Autodesk Inventor part; units mm, degrees
(part 2 of 2)
  spline S24 degree 3 poles (-2.2615, 80.5172) (-2.1729, 80.4485) (-1.9959, 80.3111) (-1.7411, 80.0916) (-1.5366, 79.9001) (-1.379, 79.7408) (-1.2639, 79.6183) (-1.1529, 79.4921) (-1.0079, 79.3211) (-0.9013, 79.1554) (-0.7866, 79.0322) (-0.7323, 78.9876) (-0.6853, 78.9569) (-0.6478, 78.9379) (-0.6091, 78.9214) (-0.5689, 78.909) (-0.5276, 78.9009) (-0.4857, 78.8971) (-0.4436, 78.8966) (-0.402, 78.903) (-0.3606, 78.9107) (-0.3079, 78.9303) (-0.2436, 78.958) (-0.1785, 78.9835) (-0.1272, 79.0065) (-0.0924, 79.0302) (-0.0583, 79.0548) (-0.0286, 79.0848) (-0.0015, 79.1169) (0.0221, 79.1518) (0.042, 79.1888) (0.058, 79.2277) (0.0713, 79.2677) (0.0832, 79.3225) (0.0904, 79.3923) (0.0854, 79.5606) (0.0448, 79.7534) (0.0277, 79.977) (0.018, 80.1448) (0.0138, 80.3128) (0.0139, 80.5369) (0.0248, 80.8169) (0.0517, 81.1521) (0.0811, 81.3743) (0.0958, 81.4854) knots 0 0 0 0 0.033613 0.067227 0.100839 0.117647 0.134454 0.151261 0.168068 0.201677 0.210077 0.218473 0.222676 0.226878 0.231076 0.235279 0.239479 0.24368 0.247882 0.252083 0.256283 0.260485 0.268889 0.277292 0.281494 0.285694 0.289895 0.294097 0.298298 0.302498 0.306701 0.310899 0.315101 0.319304 0.3277 0.3361 0.369709 0.386516 0.403323 0.420131 0.436938 0.470551 0.504164 0.537777 0.537777 0.537777 0.537777 projected
  arc A24 (-2.2615, 80.5172) -> (-2.9354, 80.1729) centre (6.5, 62.5385) ccw projected
  spline S25 degree 3 poles (-5.1012, 78.8299) (-5.0026, 78.7768) (-4.8053, 78.6704) (-4.5179, 78.4958) (-4.2846, 78.3406) (-4.1029, 78.2094) (-3.9692, 78.1075) (-3.839, 78.0012) (-3.6678, 77.8564) (-3.5354, 77.7105) (-3.4019, 77.6079) (-3.3411, 77.5728) (-3.2897, 77.5503) (-3.2496, 77.5377) (-3.2087, 77.5278) (-3.167, 77.5223) (-3.1249, 77.521) (-3.083, 77.5242) (-3.0413, 77.5306) (-3.0013, 77.5438) (-2.9618, 77.5582) (-2.9131, 77.5862) (-2.8542, 77.6241) (-2.7941, 77.66) (-2.7474, 77.6911) (-2.7169, 77.7202) (-2.6873, 77.7501) (-2.663, 77.7846) (-2.6416, 77.8207) (-2.624, 77.859) (-2.6104, 77.8988) (-2.6011, 77.9398) (-2.5946, 77.9814) (-2.5919, 78.0374) (-2.5962, 78.1075) (-2.6288, 78.2727) (-2.7006, 78.4562) (-2.7543, 78.6738) (-2.7915, 78.8377) (-2.8233, 79.0028) (-2.8601, 79.2239) (-2.8954, 79.5018) (-2.924, 79.8369) (-2.9316, 80.0609) (-2.9354, 80.1729) knots 0 0 0 0 0.033613 0.067227 0.100839 0.117647 0.134454 0.151261 0.168068 0.201677 0.210077 0.218473 0.222676 0.226878 0.231076 0.235279 0.239479 0.24368 0.247882 0.252083 0.256283 0.260485 0.268889 0.277292 0.281494 0.285694 0.289895 0.294097 0.298298 0.302498 0.306701 0.310899 0.315101 0.319304 0.3277 0.3361 0.369709 0.386516 0.403323 0.420131 0.436938 0.470551 0.504164 0.537777 0.537777 0.537777 0.537777 projected
  arc A25 (-5.1012, 78.8299) -> (-5.7093, 78.3793) centre (6.5, 62.5385) ccw projected
  spline S26 degree 3 poles (-7.6244, 76.6983) (-7.5184, 76.662) (-7.3063, 76.5896) (-6.9941, 76.4647) (-6.7384, 76.35) (-6.5377, 76.2504) (-6.389, 76.1719) (-6.243, 76.0886) (-6.0504, 75.9739) (-5.8958, 75.8518) (-5.7472, 75.7725) (-5.6814, 75.748) (-5.6271, 75.7342) (-5.5854, 75.7284) (-5.5434, 75.7254) (-5.5014, 75.7268) (-5.4597, 75.7324) (-5.4188, 75.7425) (-5.3788, 75.7557) (-5.3416, 75.7753) (-5.3049, 75.796) (-5.2615, 75.8317) (-5.2097, 75.8787) (-5.1563, 75.924) (-5.1153, 75.9624) (-5.09, 75.9961) (-5.0658, 76.0305) (-5.0475, 76.0684) (-5.0322, 76.1076) (-5.0212, 76.1483) (-5.0144, 76.1898) (-5.0119, 76.2318) (-5.0123, 76.2738) (-5.0189, 76.3295) (-5.0347, 76.398) (-5.0941, 76.5555) (-5.1951, 76.7247) (-5.2839, 76.9306) (-5.3476, 77.0861) (-5.4061, 77.2437) (-5.4788, 77.4557) (-5.5594, 77.724) (-5.6427, 78.0498) (-5.6871, 78.2695) (-5.7093, 78.3793) knots 0 0 0 0 0.033613 0.067227 0.100839 0.117647 0.134454 0.151261 0.168068 0.201677 0.210077 0.218473 0.222676 0.226878 0.231076 0.235279 0.239479 0.24368 0.247882 0.252083 0.256283 0.260485 0.268889 0.277292 0.281494 0.285694 0.289895 0.294097 0.298298 0.302498 0.306701 0.310899 0.315101 0.319304 0.3277 0.3361 0.369709 0.386516 0.403323 0.420131 0.436938 0.470551 0.504164 0.537777 0.537777 0.537777 0.537777 projected
  arc A26 (-7.6244, 76.6983) -> (-8.1501, 76.1537) centre (6.5, 62.5385) ccw projected
  spline S27 degree 3 poles (-9.7624, 74.1803) (-9.6519, 74.162) (-9.4308, 74.1255) (-9.1022, 74.0537) (-8.8312, 73.9826) (-8.6168, 73.9175) (-8.4572, 73.8645) (-8.2995, 73.8064) (-8.0906, 73.7249) (-7.918, 73.63) (-7.7585, 73.5762) (-7.6895, 73.5628) (-7.6336, 73.5582) (-7.5916, 73.5593) (-7.5497, 73.5633) (-7.5084, 73.5715) (-7.4682, 73.584) (-7.4296, 73.6006) (-7.3923, 73.6203) (-7.3588, 73.6457) (-7.326, 73.6722) (-7.2891, 73.7145) (-7.2457, 73.7694) (-7.2005, 73.8229) (-7.1664, 73.8675) (-7.147, 73.9049) (-7.1288, 73.9428) (-7.1169, 73.9833) (-7.1084, 74.0244) (-7.1042, 74.0663) (-7.1043, 74.1084) (-7.1088, 74.1502) (-7.1161, 74.1916) (-7.1317, 74.2455) (-7.1586, 74.3104) (-7.2431, 74.456) (-7.3706, 74.6063) (-7.492, 74.7947) (-7.5804, 74.9376) (-7.6641, 75.0834) (-7.7707, 75.2806) (-7.8944, 75.532) (-8.0302, 75.8396) (-8.1101, 76.049) (-8.1501, 76.1537) knots 0 0 0 0 0.033613 0.067227 0.100839 0.117647 0.134454 0.151261 0.168068 0.201677 0.210077 0.218473 0.222676 0.226878 0.231076 0.235279 0.239479 0.24368 0.247882 0.252083 0.256283 0.260485 0.268889 0.277292 0.281494 0.285694 0.289895 0.294097 0.298298 0.302498 0.306701 0.310899 0.315101 0.319304 0.3277 0.3361 0.369709 0.386516 0.403323 0.420131 0.436938 0.470551 0.504164 0.537777 0.537777 0.537777 0.537777 projected
  arc A27 (-9.7624, 74.1803) -> (-10.1913, 73.5567) centre (6.5, 62.5385) ccw projected
  spline S28 degree 3 poles (-11.4568, 71.3448) (-11.3448, 71.345) (-11.1206, 71.3453) (-10.7848, 71.3286) (-10.5057, 71.3031) (-10.2835, 71.2742) (-10.1174, 71.2482) (-9.9523, 71.2168) (-9.7329, 71.1708) (-9.547, 71.1056) (-9.3808, 71.0788) (-9.3105, 71.0769) (-9.2546, 71.0816) (-9.2133, 71.0896) (-9.1727, 71.1004) (-9.1334, 71.1153) (-9.0957, 71.1343) (-9.0604, 71.157) (-9.0268, 71.1825) (-8.9979, 71.2131) (-8.97, 71.2446) (-8.9405, 71.2924) (-8.9068, 71.3538) (-8.871, 71.4139) (-8.8447, 71.4636) (-8.8317, 71.5036) (-8.82, 71.544) (-8.815, 71.5859) (-8.8133, 71.6279) (-8.8161, 71.6699) (-8.8231, 71.7114) (-8.8344, 71.7519) (-8.8484, 71.7916) (-8.8727, 71.8421) (-8.9099, 71.9017) (-9.0172, 72.0314) (-9.1677, 72.1586) (-9.3185, 72.3245) (-9.4292, 72.451) (-9.5358, 72.581) (-9.6734, 72.7579) (-9.8367, 72.9856) (-10.0213, 73.2666) (-10.1346, 73.46) (-10.1913, 73.5567) knots 0 0 0 0 0.033613 0.067227 0.100839 0.117647 0.134454 0.151261 0.168068 0.201677 0.210077 0.218473 0.222676 0.226878 0.231076 0.235279 0.239479 0.24368 0.247882 0.252083 0.256283 0.260485 0.268889 0.277292 0.281494 0.285694 0.289895 0.294097 0.298298 0.302498 0.306701 0.310899 0.315101 0.319304 0.3277 0.3361 0.369709 0.386516 0.403323 0.420131 0.436938 0.470551 0.504164 0.537777 0.537777 0.537777 0.537777 projected
  arc A28 (-11.4568, 71.3448) -> (-11.7772, 70.6591) centre (6.5, 62.5385) ccw projected
  spline S29 degree 3 poles (-12.6614, 68.2691) (-12.5509, 68.2877) (-12.3299, 68.325) (-11.9959, 68.3637) (-11.7164, 68.3845) (-11.4925, 68.3926) (-11.3244, 68.3943) (-11.1563, 68.3905) (-10.9323, 68.3813) (-10.7382, 68.3475) (-10.5699, 68.3484) (-10.5003, 68.3582) (-10.4459, 68.372) (-10.4065, 68.3867) (-10.3682, 68.404) (-10.3319, 68.4252) (-10.2979, 68.4501) (-10.2667, 68.4783) (-10.2378, 68.509) (-10.2144, 68.5439) (-10.192, 68.5796) (-10.1708, 68.6316) (-10.1476, 68.6977) (-10.1222, 68.7629) (-10.1045, 68.8162) (-10.0982, 68.8578) (-10.0933, 68.8996) (-10.0953, 68.9417) (-10.1005, 68.9834) (-10.1102, 69.0244) (-10.1239, 69.0642) (-10.1417, 69.1023) (-10.1621, 69.1391) (-10.1944, 69.185) (-10.2409, 69.2376) (-10.3681, 69.3479) (-10.5374, 69.4486) (-10.7135, 69.5874) (-10.8435, 69.6939) (-10.97, 69.8046) (-11.1348, 69.9565) (-11.3334, 70.1541) (-11.5618, 70.401) (-11.7054, 70.5731) (-11.7772, 70.6591) knots 0 0 0 0 0.033613 0.067227 0.100839 0.117647 0.134454 0.151261 0.168068 0.201677 0.210077 0.218473 0.222676 0.226878 0.231076 0.235279 0.239479 0.24368 0.247882 0.252083 0.256283 0.260485 0.268889 0.277292 0.281494 0.285694 0.289895 0.294097 0.298298 0.302498 0.306701 0.310899 0.315101 0.319304 0.3277 0.3361 0.369709 0.386516 0.403323 0.420131 0.436938 0.470551 0.504164 0.537777 0.537777 0.537777 0.537777 projected
  arc A29 (-12.6614, 68.2691) -> (-12.8645, 67.5401) centre (6.5, 62.5385) ccw projected
  spline S30 degree 3 poles (-13.3433, 65.0371) (-13.2374, 65.0737) (-13.0255, 65.1467) (-12.7024, 65.2399) (-12.4302, 65.3065) (-12.2106, 65.3513) (-12.0451, 65.3806) (-11.8787, 65.4045) (-11.6563, 65.4323) (-11.4592, 65.431) (-11.2933, 65.4596) (-11.2263, 65.4806) (-11.175, 65.5032) (-11.1385, 65.5242) (-11.1036, 65.5476) (-11.0712, 65.5745) (-11.0418, 65.6046) (-11.0157, 65.6376) (-10.9923, 65.6726) (-10.9749, 65.7109) (-10.9587, 65.7498) (-10.9463, 65.8046) (-10.9343, 65.8736) (-10.92, 65.9421) (-10.9113, 65.9976) (-10.912, 66.0397) (-10.914, 66.0817) (-10.9229, 66.1229) (-10.9349, 66.1632) (-10.9512, 66.202) (-10.9713, 66.239) (-10.9951, 66.2736) (-11.0213, 66.3066) (-11.0607, 66.3465) (-11.1152, 66.3908) (-11.2588, 66.4786) (-11.4424, 66.5501) (-11.6389, 66.658) (-11.7847, 66.7417) (-11.9277, 66.83) (-12.1153, 66.9527) (-12.3437, 67.115) (-12.6096, 67.3209) (-12.7795, 67.467) (-12.8645, 67.5401) knots 0 0 0 0 0.033613 0.067227 0.100839 0.117647 0.134454 0.151261 0.168068 0.201677 0.210077 0.218473 0.222676 0.226878 0.231076 0.235279 0.239479 0.24368 0.247882 0.252083 0.256283 0.260485 0.268889 0.277292 0.281494 0.285694 0.289895 0.294097 0.298298 0.302498 0.306701 0.310899 0.315101 0.319304 0.3277 0.3361 0.369709 0.386516 0.403323 0.420131 0.436938 0.470551 0.504164 0.537777 0.537777 0.537777 0.537777 projected
  arc A30 (-13.3433, 65.0371) -> (-13.4236, 64.2845) centre (6.5, 62.5385) ccw projected
  spline S31 degree 3 poles (-13.4839, 61.7369) (-13.3855, 61.7904) (-13.1885, 61.8974) (-12.8852, 62.0425) (-12.6276, 62.1529) (-12.4184, 62.2332) (-12.26, 62.2894) (-12.0998, 62.3404) (-11.885, 62.4044) (-11.6904, 62.4355) (-11.5315, 62.4911) (-11.4688, 62.5229) (-11.4219, 62.5536) (-11.3894, 62.5803) (-11.3588, 62.6091) (-11.3313, 62.641) (-11.3072, 62.6755) (-11.2869, 62.7123) (-11.2696, 62.7507) (-11.2587, 62.7914) (-11.2491, 62.8324) (-11.246, 62.8885) (-11.2455, 62.9585) (-11.2427, 63.0284) (-11.2432, 63.0846) (-11.2508, 63.126) (-11.2597, 63.1671) (-11.2752, 63.2063) (-11.2937, 63.2441) (-11.3162, 63.2797) (-11.3421, 63.3128) (-11.3713, 63.3431) (-11.4025, 63.3713) (-11.448, 63.4042) (-11.509, 63.4389) (-11.6652, 63.5019) (-11.858, 63.5422) (-12.0696, 63.6163) (-12.2272, 63.6748) (-12.3828, 63.7384) (-12.588, 63.8285) (-12.84, 63.951) (-13.1361, 64.1103) (-13.3278, 64.2265) (-13.4236, 64.2845) knots 0 0 0 0 0.033613 0.067227 0.100839 0.117647 0.134454 0.151261 0.168068 0.201677 0.210077 0.218473 0.222676 0.226878 0.231076 0.235279 0.239479 0.24368 0.247882 0.252083 0.256283 0.260485 0.268889 0.277292 0.281494 0.285694 0.289895 0.294097 0.298298 0.302498 0.306701 0.310899 0.315101 0.319304 0.3277 0.3361 0.369709 0.386516 0.403323 0.420131 0.436938 0.470551 0.504164 0.537777 0.537777 0.537777 0.537777 projected
  arc A31 (-13.4839, 61.7369) -> (-13.4393, 60.9814) centre (6.5, 62.5385) ccw projected
  spline S32 degree 3 poles (-13.0795, 58.4586) (-12.9911, 58.5276) (-12.8145, 58.6655) (-12.5391, 58.8586) (-12.3033, 59.0099) (-12.1101, 59.1235) (-11.9631, 59.205) (-11.8135, 59.2817) (-11.6121, 59.3802) (-11.4254, 59.4429) (-11.2777, 59.5238) (-11.2212, 59.5655) (-11.1799, 59.6035) (-11.1523, 59.6352) (-11.1268, 59.6687) (-11.105, 59.7046) (-11.0869, 59.7426) (-11.0729, 59.7823) (-11.0621, 59.8231) (-11.0581, 59.865) (-11.0554, 59.907) (-11.0616, 59.9628) (-11.0726, 60.0319) (-11.0813, 60.1014) (-11.0911, 60.1567) (-11.1054, 60.1963) (-11.121, 60.2354) (-11.1427, 60.2715) (-11.1672, 60.3057) (-11.1952, 60.3371) (-11.2262, 60.3655) (-11.26, 60.3906) (-11.2954, 60.4133) (-11.3457, 60.4382) (-11.4116, 60.4624) (-11.576, 60.4989) (-11.7728, 60.5068) (-11.9937, 60.5451) (-12.1588, 60.5769) (-12.3227, 60.614) (-12.54, 60.6692) (-12.8087, 60.7485) (-13.127, 60.8569) (-13.3352, 60.9399) (-13.4393, 60.9814) knots 0 0 0 0 0.033613 0.067227 0.100839 0.117647 0.134454 0.151261 0.168068 0.201677 0.210077 0.218473 0.222676 0.226878 0.231076 0.235279 0.239479 0.24368 0.247882 0.252083 0.256283 0.260485 0.268889 0.277292 0.281494 0.285694 0.289895 0.294097 0.298298 0.302498 0.306701 0.310899 0.315101 0.319304 0.3277 0.3361 0.369709 0.386516 0.403323 0.420131 0.436938 0.470551 0.504164 0.537777 0.537777 0.537777 0.537777 projected
  arc A32 (-13.0795, 58.4586) -> (-12.9111, 57.7207) centre (6.5, 62.5385) ccw projected
  spline S33 degree 3 poles (-12.1409, 55.2916) (-12.0651, 55.3741) (-11.9136, 55.5393) (-11.6738, 55.775) (-11.466, 55.9631) (-11.2942, 56.107) (-11.1626, 56.2116) (-11.0277, 56.3118) (-10.8453, 56.4421) (-10.6714, 56.5347) (-10.5391, 56.6388) (-10.4902, 56.6892) (-10.4557, 56.7335) (-10.4337, 56.7693) (-10.4141, 56.8065) (-10.3984, 56.8456) (-10.3869, 56.8861) (-10.3796, 56.9275) (-10.3757, 56.9695) (-10.3786, 57.0114) (-10.3829, 57.0533) (-10.3981, 57.1074) (-10.4204, 57.1738) (-10.4404, 57.2408) (-10.4591, 57.2938) (-10.4798, 57.3305) (-10.5016, 57.3665) (-10.529, 57.3985) (-10.5587, 57.4282) (-10.5915, 57.4546) (-10.6268, 57.4775) (-10.6643, 57.4967) (-10.7029, 57.5132) (-10.7566, 57.5296) (-10.8256, 57.5426) (-10.9937, 57.5515) (-11.1892, 57.5269) (-11.4134, 57.5283) (-11.5814, 57.5325) (-11.7493, 57.5422) (-11.9726, 57.5608) (-12.2507, 57.5948) (-12.5826, 57.6493) (-12.8016, 57.6969) (-12.9111, 57.7207) knots 0 0 0 0 0.033613 0.067227 0.100839 0.117647 0.134454 0.151261 0.168068 0.201677 0.210077 0.218473 0.222676 0.226878 0.231076 0.235279 0.239479 0.24368 0.247882 0.252083 0.256283 0.260485 0.268889 0.277292 0.281494 0.285694 0.289895 0.294097 0.298298 0.302498 0.306701 0.310899 0.315101 0.319304 0.3277 0.3361 0.369709 0.386516 0.403323 0.420131 0.436938 0.470551 0.504164 0.537777 0.537777 0.537777 0.537777 projected
  arc A33 (-12.1409, 55.2916) -> (-11.8534, 54.5915) centre (6.5, 62.5385) ccw projected
  spline S34 degree 3 poles (-10.6939, 52.3222) (-10.6327, 52.4161) (-10.5104, 52.6039) (-10.3127, 52.8759) (-10.1387, 53.0956) (-9.993, 53.2658) (-9.8804, 53.3907) (-9.7638, 53.5117) (-9.6053, 53.6703) (-9.449, 53.7903) (-9.3356, 53.9148) (-9.2957, 53.9725) (-9.269, 54.0219) (-9.2531, 54.0608) (-9.2399, 54.1007) (-9.2309, 54.1418) (-9.2262, 54.1837) (-9.2259, 54.2257) (-9.2289, 54.2678) (-9.2387, 54.3087) (-9.2498, 54.3493) (-9.2737, 54.4001) (-9.3066, 54.4619) (-9.3374, 54.5248) (-9.3646, 54.5739) (-9.391, 54.6067) (-9.4184, 54.6387) (-9.4507, 54.6657) (-9.485, 54.6901) (-9.5216, 54.7108) (-9.5602, 54.7276) (-9.6003, 54.7403) (-9.6412, 54.7502) (-9.6968, 54.7575) (-9.767, 54.759) (-9.9343, 54.7401) (-10.1231, 54.6837) (-10.3445, 54.6482) (-10.5109, 54.6247) (-10.678, 54.6066) (-10.9014, 54.5882) (-11.1813, 54.5759) (-11.5176, 54.5751) (-11.7414, 54.586) (-11.8534, 54.5915) knots 0 0 0 0 0.033613 0.067227 0.100839 0.117647 0.134454 0.151261 0.168068 0.201677 0.210077 0.218473 0.222676 0.226878 0.231076 0.235279 0.239479 0.24368 0.247882 0.252083 0.256283 0.260485 0.268889 0.277292 0.281494 0.285694 0.289895 0.294097 0.298298 0.302498 0.306701 0.310899 0.315101 0.319304 0.3277 0.3361 0.369709 0.386516 0.403323 0.420131 0.436938 0.470551 0.504164 0.537777 0.537777 0.537777 0.537777 projected
  arc A34 (-10.6939, 52.3222) -> (-10.295, 51.679) centre (6.5, 62.5385) ccw projected
  spline S35 degree 3 poles (-8.7778, 49.6316) (-8.733, 49.7342) (-8.6432, 49.9396) (-8.493, 50.2405) (-8.3576, 50.4858) (-8.2418, 50.6777) (-8.1513, 50.8193) (-8.0562, 50.9579) (-7.926, 51.1404) (-7.7915, 51.2844) (-7.7003, 51.4259) (-7.6703, 51.4895) (-7.6522, 51.5425) (-7.6429, 51.5836) (-7.6365, 51.6251) (-7.6343, 51.6671) (-7.6366, 51.7092) (-7.6432, 51.7507) (-7.6531, 51.7917) (-7.6695, 51.8304) (-7.6871, 51.8687) (-7.7191, 51.9149) (-7.7617, 51.9704) (-7.8024, 52.0273) (-7.8373, 52.0714) (-7.8687, 52.0993) (-7.901, 52.1263) (-7.9374, 52.1477) (-7.9752, 52.1661) (-8.0147, 52.1805) (-8.0556, 52.1907) (-8.0972, 52.1966) (-8.1391, 52.1997) (-8.1952, 52.1978) (-8.2647, 52.1876) (-8.4266, 52.1415) (-8.6035, 52.0548) (-8.816, 51.9833) (-8.9763, 51.9327) (-9.1382, 51.8873) (-9.3555, 51.8324) (-9.6296, 51.7743) (-9.9611, 51.7181) (-10.1837, 51.692) (-10.295, 51.679) knots 0 0 0 0 0.033613 0.067227 0.100839 0.117647 0.134454 0.151261 0.168068 0.201677 0.210077 0.218473 0.222676 0.226878 0.231076 0.235279 0.239479 0.24368 0.247882 0.252083 0.256283 0.260485 0.268889 0.277292 0.281494 0.285694 0.289895 0.294097 0.298298 0.302498 0.306701 0.310899 0.315101 0.319304 0.3277 0.3361 0.369709 0.386516 0.403323 0.420131 0.436938 0.470551 0.504164 0.537777 0.537777 0.537777 0.537777 projected
  arc A35 (-8.7778, 49.6316) -> (-8.2785, 49.0628) centre (6.5, 62.5385) ccw projected
  spline S36 degree 3 poles (-6.445, 47.2929) (-6.4177, 47.4016) (-6.363, 47.619) (-6.2643, 47.9404) (-6.1711, 48.2047) (-6.0885, 48.413) (-6.0226, 48.5676) (-5.9516, 48.72) (-5.8532, 48.9214) (-5.7443, 49.0856) (-5.6775, 49.2402) (-5.6585, 49.3078) (-5.6493, 49.3631) (-5.6469, 49.4051) (-5.6474, 49.4472) (-5.6522, 49.489) (-5.6613, 49.5301) (-5.6747, 49.5699) (-5.6912, 49.6087) (-5.7137, 49.6443) (-5.7374, 49.6791) (-5.7765, 49.7194) (-5.8277, 49.7671) (-5.8772, 49.8166) (-5.9189, 49.8543) (-5.9545, 49.8767) (-5.9908, 49.898) (-6.0302, 49.9131) (-6.0705, 49.9251) (-6.1119, 49.9327) (-6.1539, 49.9361) (-6.1959, 49.935) (-6.2378, 49.9312) (-6.2927, 49.92) (-6.3596, 49.8986) (-6.5117, 49.8264) (-6.672, 49.7118) (-6.8698, 49.6063) (-7.0196, 49.53) (-7.1718, 49.4586) (-7.3771, 49.3687) (-7.6379, 49.2663) (-7.9556, 49.1563) (-8.1709, 49.0939) (-8.2785, 49.0628) knots 0 0 0 0 0.033613 0.067227 0.100839 0.117647 0.134454 0.151261 0.168068 0.201677 0.210077 0.218473 0.222676 0.226878 0.231076 0.235279 0.239479 0.24368 0.247882 0.252083 0.256283 0.260485 0.268889 0.277292 0.281494 0.285694 0.289895 0.294097 0.298298 0.302498 0.306701 0.310899 0.315101 0.319304 0.3277 0.3361 0.369709 0.386516 0.403323 0.420131 0.436938 0.470551 0.504164 0.537777 0.537777 0.537777 0.537777 projected
  arc A36 (-6.445, 47.2929) -> (-5.859, 46.8141) centre (6.5, 62.5385) ccw projected
  spline S37 degree 3 poles (-3.7592, 45.3702) (-3.7501, 45.4819) (-3.7319, 45.7053) (-3.6875, 46.0386) (-3.639, 46.3146) (-3.5919, 46.5337) (-3.5522, 46.697) (-3.5073, 46.859) (-3.4434, 47.0739) (-3.363, 47.2538) (-3.3226, 47.4172) (-3.3149, 47.487) (-3.315, 47.5431) (-3.3196, 47.5849) (-3.3269, 47.6263) (-3.3386, 47.6668) (-3.3543, 47.7058) (-3.3741, 47.7429) (-3.3967, 47.7785) (-3.4248, 47.8098) (-3.4539, 47.8402) (-3.4992, 47.8736) (-3.5575, 47.9122) (-3.6145, 47.9529) (-3.6618, 47.9832) (-3.7006, 47.9994) (-3.7399, 48.0145) (-3.7812, 48.0229) (-3.823, 48.0281) (-3.8651, 48.0288) (-3.907, 48.0252) (-3.9483, 48.0173) (-3.989, 48.0066) (-4.0413, 47.9865) (-4.1038, 47.9544) (-4.242, 47.8581) (-4.3812, 47.7187) (-4.5589, 47.5821) (-4.6941, 47.4822) (-4.8324, 47.3867) (-5.0201, 47.2643) (-5.2605, 47.1203) (-5.5558, 46.9595) (-5.7579, 46.8625) (-5.859, 46.8141) knots 0 0 0 0 0.033613 0.067227 0.100839 0.117647 0.134454 0.151261 0.168068 0.201677 0.210077 0.218473 0.222676 0.226878 0.231076 0.235279 0.239479 0.24368 0.247882 0.252083 0.256283 0.260485 0.268889 0.277292 0.281494 0.285694 0.289895 0.294097 0.298298 0.302498 0.306701 0.310899 0.315101 0.319304 0.3277 0.3361 0.369709 0.386516 0.403323 0.420131 0.436938 0.470551 0.504164 0.537777 0.537777 0.537777 0.537777 projected
  arc A37 (-3.7592, 45.3702) -> (-3.1023, 44.9943) centre (6.5, 62.5385) ccw projected
  circle A38 centre (6.5, 62.5385) radius 16 projected
  arc A39 (25.4036, 41.8198) -> (23.2102, 40.8992) centre (27.6407, 33.4167) ccw projected
  arc A40 (23.2102, 40.8992) -> (22.7103, 41.3835) centre (16.1803, 34.1432) ccw projected
  arc A41 (22.7103, 41.3835) -> (23.561, 43.6049) centre (15.0912, 45.5749) ccw projected
  arc A42 (23.561, 43.6049) -> (22.8672, 44.1074) centre (16.1803, 34.1432) ccw projected
  arc A43 (22.8672, 44.1074) -> (21.022, 42.606) centre (27.3812, 36.6749) ccw projected
  arc A44 (21.022, 42.606) -> (20.406, 42.9299) centre (16.1803, 34.1432) ccw projected
  arc A45 (20.406, 42.9299) -> (20.5964, 45.3011) centre (11.9147, 44.805) ccw projected
  arc A46 (20.5964, 45.3011) -> (19.7891, 45.5877) centre (16.1803, 34.1432) ccw projected
  arc A47 (19.7891, 45.5877) -> (18.4416, 43.6273) centre (26.2142, 39.728) ccw projected
  arc A48 (18.4416, 43.6273) -> (17.7593, 43.7645) centre (16.1803, 34.1432) ccw projected
  arc A49 (17.7593, 43.7645) -> (17.2739, 46.0932) centre (9.0837, 43.1713) ccw projected
  arc A50 (17.2739, 46.0932) -> (16.4186, 46.1408) centre (16.1803, 34.1432) ccw projected
  arc A51 (16.4186, 46.1408) -> (15.678, 43.8802) centre (24.2344, 42.3286) ccw projected
  arc A52 (15.678, 43.8802) -> (14.9847, 43.8196) centre (16.1803, 34.1432) ccw projected
  arc A53 (14.9847, 43.8196) -> (13.8629, 45.9173) centre (6.8276, 40.8063) ccw projected
  arc A54 (13.8629, 45.9173) -> (13.0289, 45.722) centre (16.1803, 34.1432) ccw projected
  arc A55 (13.0289, 45.722) -> (12.9551, 43.3443) centre (21.602, 44.2662) ccw projected
  arc A56 (12.9551, 43.3443) -> (12.307, 43.0908) centre (16.1803, 34.1432) ccw projected
  arc A57 (12.307, 43.0908) -> (10.6396, 44.7875) centre (5.3292, 37.9014) ccw projected
  arc A58 (10.6396, 44.7875) -> (9.8944, 44.3651) centre (16.1803, 34.1432) ccw projected
  arc A59 (9.8944, 44.3651) -> (10.4935, 42.063) centre (18.5304, 45.3836) ccw projected
  arc A60 (10.4935, 42.063) -> (9.943, 41.6371) centre (16.1803, 34.1432) ccw projected
  arc A61 (9.943, 41.6371) -> (7.8652, 42.7953) centre (4.71, 34.6921) ccw projected
  arc A62 (7.8652, 42.7953) -> (7.2692, 42.1801) centre (16.1803, 34.1432) ccw projected
  arc A63 (7.2692, 42.1801) -> (8.4926, 40.14) centre (15.2684, 45.5904) ccw projected
  arc A64 (8.4926, 40.14) -> (8.0844, 39.5763) centre (16.1803, 34.1432) ccw projected
  arc A65 (8.0844, 39.5763) -> (5.7645, 40.1022) centre (5.0199, 31.4383) ccw projected
  arc A66 (5.7645, 40.1022) -> (5.3659, 39.344) centre (16.1803, 34.1432) ccw projected
  arc A67 (5.3659, 39.344) -> (7.1145, 37.7312) centre (12.0803, 44.8698) ccw projected
  arc A68 (7.1145, 37.7312) -> (6.8816, 37.0753) centre (16.1803, 34.1432) ccw projected
  arc A69 (6.8816, 37.0753) -> (4.5075, 36.9264) centre (6.2341, 28.4036) ccw projected
  arc A70 (4.5075, 36.9264) -> (4.3387, 36.0865) centre (16.1803, 34.1432) ccw projected
  arc A71 (4.3387, 36.0865) -> (6.4709, 35.0318) centre (9.2244, 43.2802) ccw projected
  arc A72 (6.4709, 35.0318) -> (6.4322, 34.3368) centre (16.1803, 34.1432) ccw projected
  arc A73 (6.4322, 34.3368) -> (4.1962, 33.525) centre (8.254, 25.8339) ccw projected
  arc A74 (4.1962, 33.525) -> (4.2709, 32.6717) centre (16.1803, 34.1432) ccw projected
  arc A75 (4.2709, 32.6717) -> (6.6138, 32.2603) centre (6.9319, 40.9503) ccw projected
  arc A76 (6.6138, 32.2603) -> (6.7725, 31.5826) centre (16.1803, 34.1432) ccw projected
  arc A77 (6.7725, 31.5826) -> (4.8558, 30.1738) centre (10.916, 23.9374) ccw projected
  arc A78 (4.8558, 30.1738) -> (5.1679, 29.376) centre (16.1803, 34.1432) ccw projected
  arc A79 (5.1679, 29.376) -> (7.5318, 29.6414) centre (5.3888, 38.069) ccw projected
  arc A80 (7.5318, 29.6414) -> (7.875, 29.0359) centre (16.1803, 34.1432) ccw projected
  arc A81 (7.875, 29.0359) -> (6.4329, 27.1441) centre (14.0046, 22.8677) ccw projected
  arc A82 (6.4329, 27.1441) -> (6.957, 26.4665) centre (16.1803, 34.1432) ccw projected
  arc A83 (6.957, 26.4665) -> (9.1504, 27.3872) centre (4.7198, 34.8697) ccw projected
  arc A84 (9.1504, 27.3872) -> (9.6503, 26.9029) centre (16.1803, 34.1432) ccw projected
  arc A85 (9.6503, 26.9029) -> (8.7996, 24.6814) centre (17.2694, 22.7115) ccw projected
  arc A86 (8.7996, 24.6814) -> (9.4934, 24.179) centre (16.1803, 34.1432) ccw projected
  arc A87 (9.4934, 24.179) -> (11.3386, 25.6803) centre (4.9794, 31.6115) ccw projected
  arc A88 (11.3386, 25.6803) -> (11.9546, 25.3565) centre (16.1803, 34.1432) ccw projected
  arc A89 (11.9546, 25.3565) -> (11.7642, 22.9853) centre (20.4459, 23.4814) ccw projected
  arc A90 (11.7642, 22.9853) -> (12.5715, 22.6987) centre (16.1803, 34.1432) ccw projected
  arc A91 (12.5715, 22.6987) -> (13.919, 24.659) centre (6.1464, 28.5584) ccw projected
  arc A92 (13.919, 24.659) -> (14.6013, 24.5219) centre (16.1803, 34.1432) ccw projected
  arc A93 (14.6013, 24.5219) -> (15.0867, 22.1931) centre (23.2769, 25.115) ccw projected
  arc A94 (15.0867, 22.1931) -> (15.9419, 22.1455) centre (16.1803, 34.1432) ccw projected
  arc A95 (15.9419, 22.1455) -> (16.6826, 24.4061) centre (8.1262, 25.9577) ccw projected
  arc A96 (16.6826, 24.4061) -> (17.3759, 24.4668) centre (16.1803, 34.1432) ccw projected
  arc A97 (17.3759, 24.4668) -> (18.4977, 22.3691) centre (25.533, 27.4801) ccw projected
  arc A98 (18.4977, 22.3691) -> (19.3317, 22.5644) centre (16.1803, 34.1432) ccw projected
  arc A99 (19.3317, 22.5644) -> (19.4055, 24.942) centre (10.7586, 24.0202) ccw projected
  arc A100 (19.4055, 24.942) -> (20.0536, 25.1956) centre (16.1803, 34.1432) ccw projected
  arc A101 (20.0536, 25.1956) -> (21.721, 23.4989) centre (27.0313, 30.3849) ccw projected
  arc A102 (21.721, 23.4989) -> (22.4662, 23.9213) centre (16.1803, 34.1432) ccw projected
  arc A103 (22.4662, 23.9213) -> (21.8671, 26.2234) centre (13.8302, 22.9028) ccw projected
  arc A104 (21.8671, 26.2234) -> (22.4176, 26.6493) centre (16.1803, 34.1432) ccw projected
  arc A105 (22.4176, 26.6493) -> (24.4954, 25.491) centre (27.6506, 33.5943) ccw projected
  arc A106 (24.4954, 25.491) -> (25.0914, 26.1063) centre (16.1803, 34.1432) ccw projected
  arc A107 (25.0914, 26.1063) -> (23.868, 28.1463) centre (17.0922, 22.696) ccw projected
  arc A108 (23.868, 28.1463) -> (24.2762, 28.7101) centre (16.1803, 34.1432) ccw projected
  arc A109 (24.2762, 28.7101) -> (26.5961, 28.1841) centre (27.3406, 36.8481) ccw projected
  arc A110 (26.5961, 28.1841) -> (26.9947, 28.9424) centre (16.1803, 34.1432) ccw projected
  arc A111 (26.9947, 28.9424) -> (25.2461, 30.5551) centre (20.2803, 23.4166) ccw projected
  arc A112 (25.2461, 30.5551) -> (25.4789, 31.211) centre (16.1803, 34.1432) ccw projected
  arc A113 (25.4789, 31.211) -> (27.8531, 31.36) centre (26.1265, 39.8827) ccw projected
  arc A114 (27.8531, 31.36) -> (28.0219, 32.1998) centre (16.1803, 34.1432) ccw projected
  arc A115 (28.0219, 32.1998) -> (25.8897, 33.2546) centre (23.1362, 25.0062) ccw projected
  arc A116 (25.8897, 33.2546) -> (25.9284, 33.9495) centre (16.1803, 34.1432) ccw projected
  arc A117 (25.9284, 33.9495) -> (28.1644, 34.7613) centre (24.1066, 42.4524) ccw projected
  arc A118 (28.1644, 34.7613) -> (28.0897, 35.6147) centre (16.1803, 34.1432) ccw projected
  arc A119 (28.0897, 35.6147) -> (25.7468, 36.026) centre (25.4287, 27.336) ccw projected
  arc A120 (25.7468, 36.026) -> (25.5881, 36.7037) centre (16.1803, 34.1432) ccw projected
  arc A121 (25.5881, 36.7037) -> (27.5048, 38.1126) centre (21.4446, 44.3489) ccw projected
  arc A122 (27.5048, 38.1126) -> (27.1927, 38.9104) centre (16.1803, 34.1432) ccw projected
  arc A123 (27.1927, 38.9104) -> (24.8288, 38.645) centre (26.9718, 30.2173) ccw projected
  arc A124 (24.8288, 38.645) -> (24.4856, 39.2505) centre (16.1803, 34.1432) ccw projected
  arc A125 (24.4856, 39.2505) -> (25.9277, 41.1423) centre (18.356, 45.4186) ccw projected
  arc A126 (25.9277, 41.1423) -> (25.4036, 41.8198) centre (16.1803, 34.1432) ccw projected
  arc A127 (11.7246, 16.8961) -> (10.2227, 15.407) centre (14.2615, 12.8353) ccw projected
  arc A128 (10.2227, 15.407) -> (10.7174, 14.6349) centre (15.375, 18.1635) ccw projected
  arc A129 (10.7174, 14.6349) -> (12.6979, 15.377) centre (10.0692, 19.3789) ccw projected
  arc A130 (12.6979, 15.377) -> (13.1667, 14.9925) centre (15.375, 18.1635) ccw projected
  arc A131 (13.1667, 14.9925) -> (12.8269, 12.905) centre (17.606, 13.1984) ccw projected
  arc A132 (12.8269, 12.905) -> (13.6809, 12.5712) centre (15.375, 18.1635) ccw projected
  arc A133 (13.6809, 12.5712) -> (14.847, 14.3356) centre (10.3681, 16.0281) ccw projected
  arc A134 (14.847, 14.3356) -> (15.4523, 14.3001) centre (15.375, 18.1635) ccw projected
  arc A135 (15.4523, 14.3001) -> (16.4044, 12.4116) centre (20.0983, 15.458) ccw projected
  arc A136 (16.4044, 12.4116) -> (17.2915, 12.6434) centre (15.375, 18.1635) ccw projected
  arc A137 (17.2915, 12.6434) -> (17.1978, 14.7563) centre (12.5794, 13.493) ccw projected
  arc A138 (17.1978, 14.7563) -> (17.7084, 15.0834) centre (15.375, 18.1635) ccw projected
  arc A139 (17.7084, 15.0834) -> (19.5887, 14.1152) centre (20.7864, 18.751) ccw projected
  arc A140 (19.5887, 14.1152) -> (20.1701, 14.8242) centre (15.375, 18.1635) ccw projected
  arc A141 (20.1701, 14.8242) -> (18.8524, 16.4784) centre (15.8586, 12.7418) ccw projected
  arc A142 (18.8524, 16.4784) -> (19.0731, 17.0432) centre (15.375, 18.1635) ccw projected
  arc A143 (19.0731, 17.0432) -> (21.1635, 17.365) centre (19.4076, 21.8195) ccw projected
  arc A144 (21.1635, 17.365) -> (21.2171, 18.2804) centre (15.375, 18.1635) ccw projected
  arc A145 (21.2171, 18.2804) -> (19.1787, 18.8442) centre (18.953, 14.0615) ccw projected
  arc A146 (19.1787, 18.8442) -> (19.0254, 19.4308) centre (15.375, 18.1635) ccw projected
  arc A147 (19.0254, 19.4308) -> (20.5273, 20.9199) centre (16.4885, 23.4916) ccw projected
  arc A148 (20.5273, 20.9199) -> (20.0326, 21.692) centre (15.375, 18.1635) ccw projected
  arc A149 (20.0326, 21.692) -> (18.0521, 20.9499) centre (20.6808, 16.948) ccw projected
  arc A150 (18.0521, 20.9499) -> (17.5833, 21.3344) centre (15.375, 18.1635) ccw projected
  arc A151 (17.5833, 21.3344) -> (17.9231, 23.4219) centre (13.144, 23.1285) ccw projected
  arc A152 (17.9231, 23.4219) -> (17.0691, 23.7558) centre (15.375, 18.1635) ccw projected
  arc A153 (17.0691, 23.7558) -> (15.903, 21.9913) centre (20.3819, 20.2988) ccw projected
  arc A154 (15.903, 21.9913) -> (15.2977, 22.0268) centre (15.375, 18.1635) ccw projected
  arc A155 (15.2977, 22.0268) -> (14.3456, 23.9153) centre (10.6517, 20.8689) ccw projected
  arc A156 (14.3456, 23.9153) -> (13.4585, 23.6835) centre (15.375, 18.1635) ccw projected
  arc A157 (13.4585, 23.6835) -> (13.5522, 21.5706) centre (18.1706, 22.8339) ccw projected
  arc A158 (13.5522, 21.5706) -> (13.0416, 21.2435) centre (15.375, 18.1635) ccw projected
  arc A159 (13.0416, 21.2435) -> (11.1613, 22.2118) centre (9.9636, 17.5759) ccw projected
  arc A160 (11.1613, 22.2118) -> (10.5799, 21.5027) centre (15.375, 18.1635) ccw projected
  arc A161 (10.5799, 21.5027) -> (11.8976, 19.8485) centre (14.8914, 23.5851) ccw projected
  arc A162 (11.8976, 19.8485) -> (11.6769, 19.2837) centre (15.375, 18.1635) ccw projected
  arc A163 (11.6769, 19.2837) -> (9.5865, 18.9619) centre (11.3424, 14.5074) ccw projected
  arc A164 (9.5865, 18.9619) -> (9.5329, 18.0465) centre (15.375, 18.1635) ccw projected
  arc A165 (9.5329, 18.0465) -> (11.5713, 17.4827) centre (11.797, 22.2654) ccw projected
  arc A166 (11.5713, 17.4827) -> (11.7246, 16.8961) centre (15.375, 18.1635) ccw projected
  circle A167 centre (23.5, 78.5385) radius 3.5
  circle A168 centre (5, 20) radius 3.5
  line L0 (29.5, 0) -> (29.5, 88.5385) projected
  line L1 (0, 88.5385) -> (29.5, 88.5385) projected
  circle A169 centre (23.5, 78.5385) radius 1.5
  line L2 (0, 88.5385) -> (0, 0) projected
  circle A170 centre (5, 20) radius 1.5
  line L3 (0, 0) -> (29.5, 0) projected
  circle A171 centre (16.1803, 34.1432) radius 2 projected
  point P0 (0, -0.9615)
  dimension "d7" = 7
  dimension "d11" = 7
  dimension "d12" = 6
  dimension "d13" = 10
  dimension "d14" = 3
  dimension "d15" = 5
  dimension "d16" = 3
  dimension "d17" = 20
  constraints: 4 centre point, 4 coincident
  measures "d7" diameter of A168
  measures "d11" diameter of A167
  measures "d12" distance from line of L0 A167.centre
  measures "d13" distance from line of L1 A167.centre
  measures "d14" diameter of A169
  measures "d15" distance from line of A168.centre L2
  measures "d16" diameter of A170
  measures "d17" distance from line of L3 A168.centre
hole "Hole1" at (-22.5, 79.5, 23.5) at (-22.5, 20.9615, 5) direction (1, 0, 0) diameter 3.6 end through all countersink diameter 6.7 countersink angle 90 clearance for "Countersunk Flat Head Screw ISO 2009/7046" size "M3" standard "ISO"
sketch "Sketch7" plane through (-22.5, 0.9615, 29.5) normal (0, 0, 1) x (1, 0, 0)
  line L0 (0, 11.7202) -> (0, 24.6067) projected
  line L1 (0, 56.8885) -> (0, 68.1885) projected
  line L2 (1.55, 80.3385) -> (1.55, 76.7385) projected
  line L3 (6, 24.6067) -> (6, 11.7202) projected
  line L4 (0, 11.7202) -> (6, 11.7202)
  line L5 (6, 11.7202) -> (6, 24.6067)
  line L6 (6, 24.6067) -> (0, 24.6067)
  line L7 (0, 24.6067) -> (0, 11.7202)
  line L8 (6, 0) -> (6, 88.5385) projected
  line L9 (0, 56.8885) -> (6, 56.8885)
  line L10 (6, 56.8885) -> (6, 68.1885)
  line L11 (6, 68.1885) -> (0, 68.1885)
  line L12 (0, 68.1885) -> (0, 56.8885)
  line L13 (0, 88.5385) -> (0, 0) projected
  line L14 (6, 80.3385) -> (1.55, 80.3385) projected
  line L15 (0, 76.7385) -> (6, 76.7385)
  line L16 (6, 76.7385) -> (6, 80.3385)
  line L17 (6, 80.3385) -> (0, 80.3385)
  line L18 (0, 80.3385) -> (0, 76.7385)
  line L19 (0, 11.7202) -> (6, 0)
  line L20 (6, 11.7202) -> (0, 0)
  line L21 (6, 24.6067) -> (0, 56.8885)
  line L22 (0, 24.6067) -> (6, 56.8885)
  line L23 (6, 68.1885) -> (0, 76.7385)
  line L24 (0, 68.1885) -> (6, 76.7385)
  point P0 (22.5, -0.9615)
  point P1 (3, 72.4635)
  point P2 (3, 40.7476)
  point P3 (3, 5.8601)
  constraints: 36 end point, 6 parallel, 5 point on line, 3 horizontal, 3 midpoint, 3 perpendicular, 2 other
hole "Hole2" at (-19.5, 73.425, 29.5) at (-19.5, 41.7091, 29.5) at (-19.5, 6.8216, 29.5) direction (0, 0, -1) diameter 3.6 end through all countersink diameter 6.6 countersink angle 90 clearance for "Countersunk Flat Head Screw ISO 2009/7046" size "M3" standard "ISO"
sketch "Sketch8" plane through (-22.5, 89.5, 0) normal (0, 1, 0) x (1, 0, 0)
  line L0 (0, -29.5) -> (6, -29.5) projected
  line L1 (6, 0) -> (6, -29.5) projected
  line L2 (6, 0) -> (0, 0) projected
  line L3 (0, 0) -> (0, -29.5) projected
  line L4 (0, 0) -> (0, -29.5) projected
  line L5 (0, -14.75) -> (6, -29.5)
  line L6 (6, -29.5) -> (6, -15.375)
  line L7 (6, -8.9317) -> (6, -21.8183) projected
  line L8 (0, 0) -> (6, 0) projected
  line L9 (6, -15.375) -> (0, 0)
  line L10 (0, 0) -> (0, -14.75)
  point P0 (22.5, 0)
  point P1 (3, -7.6875)
  point P2 (3, -22.125)
  constraints: 8 end point, 4 midpoint, 1 parallel
hole "Hole3" at (-19.5, 89.5, 7.6875) at (-19.5, 89.5, 22.125) direction (0, -1, 0) diameter 4 depth 3.75 counterbore diameter 4.6 counterbore depth 0.75
sketch "Sketch9" plane through (-16.5, 0.9615, 0) normal (1, 0, 0) x (0, 0, -1)
  circle A0 centre (-16.1803, 34.1432) radius 2 projected
  point P0 (0, -0.9615)
extrude "Extrusion3" cut sketch "Sketch9" against normal blind 4
body "Solid1"
